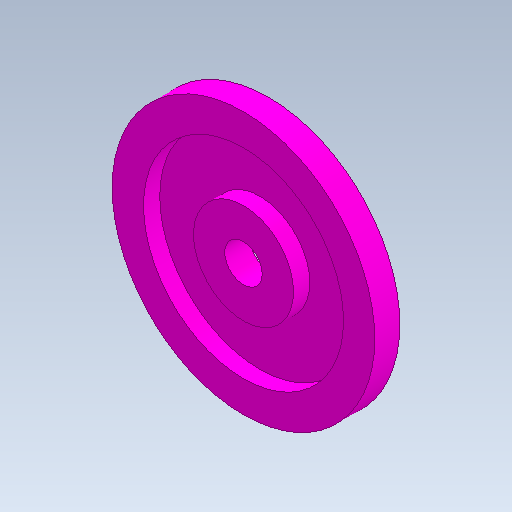
# Autodesk Inventor part: ウィング引っ掛け
Saved by Autodesk Inventor 2020.2 (Build 242310000, 310)
## iProperties
Created: 2020-04-18
Part Number: ウィング引っ掛け
Material: ポリカーボネート、スモーク
Document SubType Name: Modeling
Designer: aoyama
Mass: 0.579058 g
Surface Area: 9.27398 cm^2
Volume: 0.482549 cm^3
Density: 1.2 g/cm^3
Appearance: マゼンタ
Author: aoyama
Autodesk Inventor part; units mm, degrees
ref_plane "YZ Plane" through (0, 0, 0) normal (1, 0, 0) x (0, 1, 0)
ref_plane "XZ Plane" through (0, 0, 0) normal (0, 1, 0) x (-1, 0, 0)
ref_plane "XY Plane" through (0, 0, 0) normal (0, 0, 1) x (1, 0, 0)
sketch "スケッチ1" plane through (0, 0, 0) normal (0, 0, 1) x (1, 0, 0)
  circle A0 centre (0, 0) radius 1.5
  circle A1 centre (0, 0) radius 10.5
  dimension "d0" = 3
  dimension "d1" = 21
  constraints: 2 centre point, 2 coincident
  measures "d0" diameter of A0
  measures "d1" diameter of A1
extrude "押し出し1" add sketch "スケッチ1" along normal blind 2
sketch "スケッチ2" plane through (0, 0, 2) normal (0, 0, 1) x (1, 0, 0)
  circle A0 centre (0, 0) radius 10.5 projected
  circle A1 centre (0, 0) radius 1.5 projected
  circle A2 centre (0, 0) radius 8
  circle A3 centre (0, 0) radius 4
  dimension "d4" = 2.5
  dimension "d5" = 2.5
  dimension "d6" = 4
  constraints: 2 centre point
  measures "d4" radial gap between concentric circles of A0 A2
  measures "d5" radial gap between concentric circles of A1 A3
  measures "d6" radial gap between concentric circles of A3 A2
extrude "押し出し2" cut sketch "スケッチ2" against normal blind 1.3 contours A2
